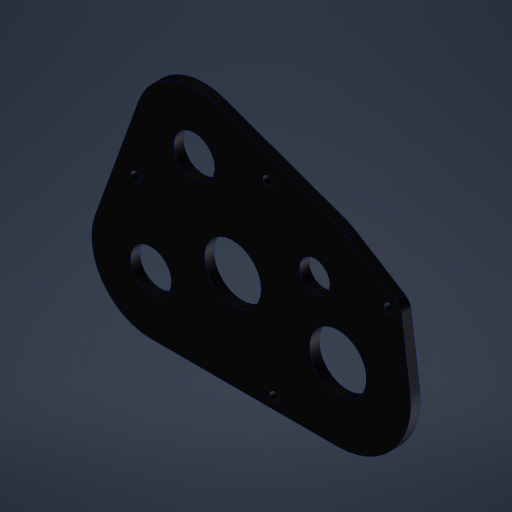
# Autodesk Inventor part: bottomplate_gearbox4
Saved by Autodesk Inventor 2024 (Build 280153000, 153)
## iProperties
Created: 2024-12-24
Part Number: bottomplate_gearbox4
Material: Aluminum 6061
Document SubType Name: Modeling
Designer: Danielle
Density: 2.7 g/cm^3
Appearance: Aluminum - Flat
Author: Danielle
Autodesk Inventor part; units mm, degrees
ref_plane "YZ Plane" through (0, 0, 0) normal (1, 0, 0) x (0, 1, 0)
ref_plane "XZ Plane" through (0, 0, 0) normal (0, 1, 0) x (-1, 0, 0)
ref_plane "XY Plane" through (0, 0, 0) normal (0, 0, 1) x (1, 0, 0)
sketch "Sketch1" plane through (0, 0, 0) normal (0, 0, 1) x (1, 0, 0)
  circle A0 centre (0, 0) radius 38.1 construction
  circle A1 centre (-41.3753, -19.4526) radius 7.62 construction
  circle A2 centre (-19.4526, 41.3753) radius 7.62 construction
  circle A3 centre (41.3753, 19.4526) radius 7.62
  circle A4 centre (-41.3753, -19.4526) radius 29.972 construction
  circle A5 centre (-19.4526, 41.3753) radius 29.972 construction
  circle A6 centre (41.3753, 19.4526) radius 29.972 construction
  line L0 (-31.2131, 8.7441) -> (-29.6148, 13.1787) construction
  line L1 (8.7441, 31.2131) -> (13.1787, 29.6148) construction
  circle A7 centre (0, 0) radius 19.05 construction
  circle A8 centre (53.1378, -12.5946) radius 35.56 construction
  circle A9 centre (53.1378, -12.5946) radius 14.2875
  circle A10 centre (41.3753, 19.4526) radius 10.3251 construction
  line L2 (44.9329, 9.7597) -> (48.2149, 0.818) construction
  circle A11 centre (53.1378, -12.5946) radius 36.83 construction
  line L3 (-41.3753, -49.4246) -> (53.1378, -49.4246)
  circle A12 centre (-19.4526, 41.3753) radius 10.3251
  circle A13 centre (-41.3753, -19.4526) radius 10.3251
  circle A14 centre (21.029, -43.7899) radius 6.35 construction
  circle A15 centre (0, 0) radius 40.64 construction
  line L4 (-7.2269, -37.4083) -> (-7.7087, -39.9022) construction
  circle A16 centre (21.029, -43.7899) radius 2.4892
  line L5 (18.2801, -38.0657) -> (17.5929, -36.6347) construction
  line L6 (25.5834, -39.365) -> (26.722, -38.2588) construction
  circle A17 centre (-49.0395, 17.6741) radius 6.35 construction
  circle A18 centre (-49.0395, 17.6741) radius 2.4892
  circle A19 centre (17.6741, 49.0395) radius 6.35 construction
  circle A20 centre (17.6741, 49.0395) radius 2.4892
  circle A21 centre (79.0191, 23.9334) radius 2.4892
  circle A22 centre (79.0191, 23.9334) radius 6.35 construction
  line L7 (-47.7557, 11.4552) -> (-47.4347, 9.9005) construction
  line L8 (-44.0835, 21.6442) -> (-42.8445, 22.6367) construction
  line L9 (11.4552, 47.7557) -> (9.9005, 47.4347) construction
  line L10 (21.6442, 44.0835) -> (22.6367, 42.8445) construction
  line L11 (72.7136, 23.1828) -> (71.1372, 22.9952) construction
  line L12 (75.348, 18.7521) -> (74.4302, 17.4568) construction
  line L13 (-69.5719, -9.2903) -> (-47.6492, 51.5375)
  arc A23 (-69.5719, -9.2903) -> (-41.3753, -49.4246) centre (-41.3753, -19.4526) ccw
  line L14 (-9.2903, 69.5719) -> (51.5375, 47.6492)
  arc A24 (-9.2903, 69.5719) -> (-47.6492, 51.5375) centre (-19.4526, 41.3753) ccw
  line L15 (57.1496, 44.9377) -> (82.3611, 29.3328)
  line L16 (85.3134, 24.7723) -> (89.645, -7.7291)
  arc A25 (57.1496, 44.9377) -> (51.5375, 47.6492) centre (41.3753, 19.4526) ccw
  arc A26 (85.3134, 24.7723) -> (82.3611, 29.3328) centre (79.0191, 23.9334) ccw
  arc A27 (53.1378, -49.4246) -> (89.645, -7.7291) centre (53.1378, -12.5946) ccw
  circle A28 centre (0, 0) radius 14.2875
  dimension "d0" = 76.2
  dimension "d5" = 28.575
  dimension "d6" = 20.6502
  dimension "d1" = 15.24
  dimension "d2" = 59.944
  dimension "d3" = 38.1
  dimension "d4" = 71.12
  dimension "d8" = 9.525
  dimension "d9" = 73.66
  dimension "d10" = 2.54
  dimension "d12" = 12.7
  dimension "d13" = 4.9784
  dimension "d14" = 1.5875
  dimension "d15" = 12.7
  dimension "d16" = 4.9784
  dimension "d17" = 12.7
  dimension "d18" = 4.9784
  dimension "d19" = 12.7
  dimension "d20" = 4.9784
  dimension "d21" = 1.5875
  dimension "d22" = 1.5875
  dimension "d23" = 1.5875
  dimension "d24" = 1.5875
  constraints: 42 point on circle, 34 end point, 26 centre point, 22 point on line, 15 coincident, 15 tangent, 5 equal radius, 4 concentric, 4 equal length, 1 horizontal, 1 line through centre, 1 perpendicular, 15 other
  measures "d1" diameter of A1
  measures "d2" diameter of A4
  measures "d3" diameter of A7
  measures "d4" diameter of A8
  measures "d8" distance of L2.start L2.end
  measures "d9" diameter of A11
  measures "d10" distance of L4.start L4.end
  measures "d12" diameter of A14
  measures "d13" diameter of A16
  measures "d14" distance of L5.start L5.end
  measures "d15" diameter of A17
  measures "d16" diameter of A18
  measures "d17" diameter of A19
  measures "d18" diameter of A20
  measures "d19" diameter of A22
  measures "d20" diameter of A21
  measures "d21" distance of L8.start L8.end
  measures "d22" distance of L7.start L7.end
  measures "d23" distance of L9.start L9.end
  measures "d24" distance of L10.start L10.end
extrude "Extrusion1" add sketch "Sketch1" along normal blind 4.7625
body "Solid1"
